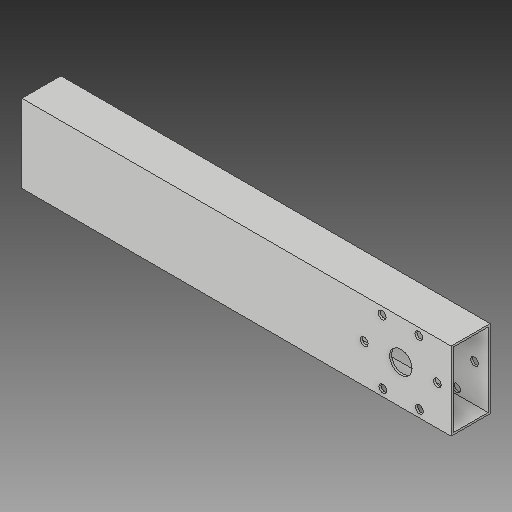
# Autodesk Inventor part: Aluminum grabber mount
Saved by Autodesk Inventor 2019 (Build 230136000, 136)
## iProperties
Created: 2019-02-04
Part Number: Aluminum grabber mount
Material: Generic
Document SubType Name: Modeling
Designer: josh
Density: 1 g/cm^3
Appearance: Default
Author: josh
Autodesk Inventor part; units mm, degrees
ref_plane "YZ Plane" through (0, 0, 0) normal (1, 0, 0) x (0, 1, 0)
ref_plane "XZ Plane" through (0, 0, 0) normal (0, 1, 0) x (-1, 0, 0)
ref_plane "XY Plane" through (0, 0, 0) normal (0, 0, 1) x (1, 0, 0)
sketch "Sketch1" plane through (0, 0, 0) normal (1, 0, 0) x (0, 1, 0)
  line L0 (0, 0) -> (50.8, 0)
  line L1 (50.8, 0) -> (50.8, -25.4)
  line L2 (50.8, -25.4) -> (0, -25.4)
  line L3 (0, -25.4) -> (0, 0)
  line L4 (49.53, -1.27) -> (1.27, -1.27)
  line L5 (1.27, -1.27) -> (1.27, -24.13)
  line L6 (1.27, -24.13) -> (49.53, -24.13)
  line L7 (49.53, -24.13) -> (49.53, -1.27)
  dimension "d0" = 50.8
  dimension "d1" = 25.4
  dimension "d2" = 1.27
  constraints: 16 end point, 4 parallel, 2 perpendicular, 1 horizontal, 3 other
  measures "d0" distance of L1.end L2.end
  measures "d1" distance of L0.end L1.end
  measures "d2" distance between parallel lines of L0 L4
extrude "Extrusion1" add sketch "Sketch1" along normal blind 279.4
sketch "Sketch2" plane through (0, 0, 0) normal (0, 0, 1) x (1, 0, 0)
  circle A0 centre (246.6677, 25.4) radius 7.3323
  point P0 (0, 0)
  constraints: 1 centre point
extrude "Extrusion2" cut sketch "Sketch2" against normal through all
sketch "Sketch3" plane through (279.4, 49.53, -1.27) normal (0, 0, -1) x (-1, 0, 0)
  circle A0 centre (8.9208, -23.9155) radius 2.5908
  circle A1 centre (21.0377, -3.4163) radius 2.5908
  circle A2 centre (20.6153, -44.6586) radius 2.5908
  circle A3 centre (56.5433, -24.4032) radius 2.5908
  circle A4 centre (44.4265, -44.9024) radius 2.5908
  circle A5 centre (44.8489, -3.6601) radius 2.5908
  point P0 (279.4, -49.53)
  constraints: 6 centre point, 12 other
extrude "Extrusion3" cut sketch "Sketch3" along normal through all both and the other way through all
body "Solid1"
